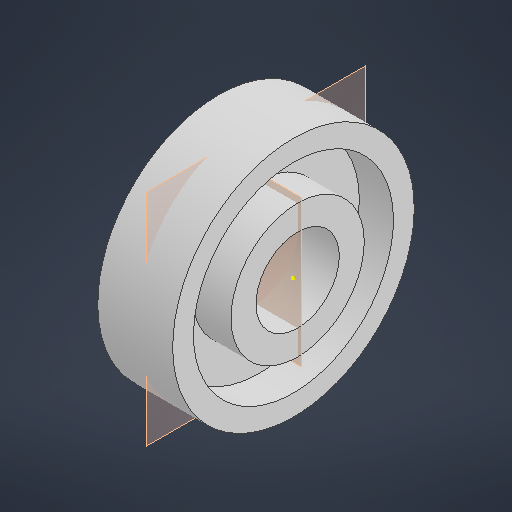
# Autodesk Inventor part: DiscoPaleSatdio1-3
Saved by Autodesk Inventor 2026.2 (Build 302298010, 298A)
## iProperties
Created: 2026-04-19
Part Number: DiscoPaleSatdio1-3
Material: Generic
Document SubType Name: Modeling
Designer: Yan
Density: 1 g/cm^3
Appearance: Default
Author: Yan
Autodesk Inventor part; units mm, degrees
ref_plane "XZ Plane" through (0, 0, 0) normal (0, 1, 0) x (-1, 0, 0)
sketch "Sketch1" plane through (0, 0, 0) normal (1, 0, 0) x (0, 1, 0)
  circle A0 centre (0, 0) radius 50
  circle A1 centre (0, 0) radius 80
  dimension "d0" = 100
  dimension "d1" = 160
  constraints: 2 centre point, 2 coincident
  measures "d0" diameter of A0
  measures "d1" diameter of A1
extrude "Extrusion1" add sketch "Sketch1" along normal blind 100
ref_plane "Work Plane1" through (0, 0, 0) normal (0, 0, 1) x (1, 0, 0)
sketch "Sketch2" plane through (0, 0, 0) normal (0, 0, 1) x (1, 0, 0)
  line L0 (0, 80) -> (100, 80) projected
  line L1 (54, 80) -> (54, 120)
  line L2 (54, 120) -> (46, 120)
  line L3 (46, 120) -> (46, 80)
  line L4 (0, -80) -> (0, 80) projected
  line L5 (-20, 0) -> (120, 0) projected
  point P0 (0, 0)
  dimension "d5" = 8
  dimension "d6" = 46
  dimension "d7" = 40
  constraints: 6 end point, 2 perpendicular, 2 point on line, 1 vertical
  measures "d5" distance between parallel lines of L3 L1
  measures "d6" distance between parallel lines of L4 L3
  measures "d7" distance between parallel lines of L0 L2
revolve "Revolution1" add sketch "Sketch2" angle 360 about axis through (-10, 0, 0) along (1, 0, 0)
ref_plane "Work Plane2" through (50, 0, 0) normal (1, 0, 0) x (0, 1, 0)
sketch "Sketch4" plane through (50, 0, 0) normal (1, 0, 0) x (0, 1, 0)
  circle A0 centre (0, 0) radius 145
  circle A1 centre (0, 0) radius 120
  dimension "d12" = 290
  dimension "d13" = 240
  constraints: 2 centre point, 2 coincident
  measures "d12" diameter of A0
  measures "d13" diameter of A1
extrude "Extrusion2" add sketch "Sketch4" along normal mid plane 90
sketch "Sketch5" plane through (95, 0, 0) normal (1, 0, 0) x (0, 0, -1)
  point P0 (0, 0)
body "Solid1"
